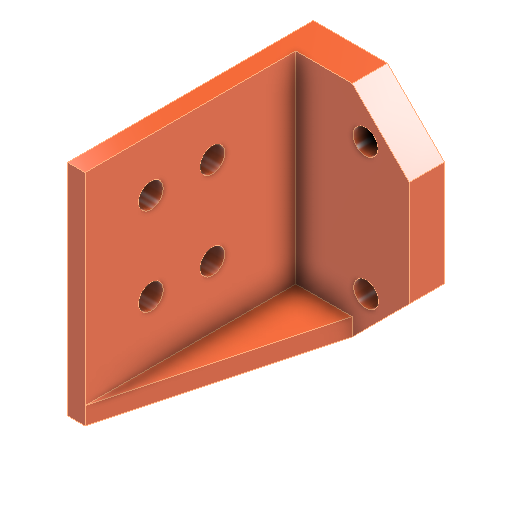
# Autodesk Inventor part: Drag Chain Base
Saved by Autodesk Inventor 2023.2 (Build 272271000, 271)
## iProperties
Created: 2023-02-07
Part Number: Drag Chain Base
Material: ABS Plastic
Document SubType Name: Modeling
Designer: remop
Density: 1.06 g/cm^3
Appearance: Smooth - Light Orange
Author: remop
Autodesk Inventor part; units mm, degrees
ref_plane "YZ Plane" through (0, 0, 0) normal (1, 0, 0) x (0, 1, 0)
ref_plane "XZ Plane" through (0, 0, 0) normal (0, 1, 0) x (-1, 0, 0)
ref_plane "XY Plane" through (0, 0, 0) normal (0, 0, 1) x (1, 0, 0)
sketch "Sketch1" plane through (0, 0, 0) normal (0, 0, 1) x (1, 0, 0)
  circle A0 centre (-45.0744, 20) radius 1.4 projected
  circle A1 centre (-45, 5.0002) radius 1.4 projected
  line L0 (-55, 0) -> (-55, 35) projected
  line L1 (-55, 25) -> (-46.5743, 25)
  line L2 (-46.5743, 25) -> (-40.0744, 18.5001)
  line L3 (-40.0744, 18.5001) -> (-40.0744, 6.5001)
  line L4 (-40.0744, 6.5001) -> (-46.5743, 0.0002)
  line L5 (-46.5743, 0.0002) -> (-55, 0.0002)
  point P0 (0, 0)
  point P1 (-50.7872, 0.0002)
  dimension "d0" = 5
  dimension "d1" = 5
  dimension "d2" = 45
  dimension "d3" = 5
  dimension "d4" = 12
  constraints: 10 end point, 4 perpendicular, 2 point on line, 1 horizontal, 1 midpoint
  measures "d0" distance from line of L1 A0.centre
  measures "d1" distance from line of L3 A0.centre
  measures "d2" angle of L2 L1
  measures "d3" vertical distance of A1.centre point (-50.787, 0)
  measures "d4" distance of L2.end L3.end
extrude "Extrusion1" add sketch "Sketch1" along normal blind 4
sketch "Sketch2" plane through (-55, 0.0002, 0) normal (-1, 0, 0) x (0, 0, 1)
  line L0 (0, 24.9998) -> (0, 0) projected
  line L1 (0, 0) -> (4, 0) projected
  line L2 (4, 24.9998) -> (4, 0) projected
  line L3 (0, 24.9998) -> (4, 24.9998) projected
  line L4 (4, 18.4999) -> (4, 24.9998) projected
  line L5 (4, 24.9998) -> (28, 24.9998)
  line L6 (28, 24.9998) -> (28, 0)
  line L7 (4, 24.9998) -> (4, 0) projected
  line L8 (28, 0) -> (4, 0)
  point P0 (0, -0.0002)
  dimension "d7" = 24
  constraints: 6 end point, 2 perpendicular, 1 horizontal
  measures "d7" distance of L2.start L5.end
extrude "Extrusion2" add sketch "Sketch2" against normal blind 2 contours L5 L6 L8 L2
sketch "Sketch4" plane through (-55, 0.0002, 0) normal (0, -1, 0) x (1, 0, 0)
  line L0 (2, 28) -> (2, 4) projected
  line L1 (2, 4) -> (8.4257, 4) projected
  line L2 (8.4257, 0) -> (8.4257, 4) projected
  line L3 (2, 4) -> (2, 28) projected
  line L4 (8.4257, 4) -> (2, 28)
  point P0 (55, 0)
  constraints: 2 end point
extrude "Extrusion4" add sketch "Sketch4" against normal blind 2
sketch "Sketch5" plane through (-55, 0.0002, 0) normal (-1, 0, 0) x (0, 0, 1)
  line L0 (0, 24.9998) -> (0, 0) projected
  line L1 (0, 0) -> (28, 0) projected
  line L2 (28, 0) -> (28, 24.9998) projected
  line L3 (0, 24.9998) -> (28, 24.9998) projected
  point P0 (0, -0.0002)
  point P1 (20.5, 19)
  point P2 (20.5, 9)
  point P3 (13.5, 9)
  point P4 (13.5, 19)
  dimension "d14" = 9
  dimension "d15" = 7
  dimension "d16" = 10
  dimension "d17" = 7.5
  constraints: 2 horizontal alignment, 2 vertical alignment
  measures "d14" distance from line of L1 point (20.5, 9)
  measures "d15" distance of point (20.5, 9) point (13.5, 9)
  measures "d16" distance of point (20.5, 19) point (20.5, 9)
  measures "d17" distance from line of L2 point (20.5, 19)
hole "Hole1" at (-55, 19.0002, 20.5) at (-55, 9.0002, 20.5) at (-55, 9.0002, 13.5) at (-55, 19.0002, 13.5) direction (1, 0, 0) diameter 2.8 end through all
equation "\"d1\" = d0"
equation "\"d3\" = d0"
body "Solid1"
